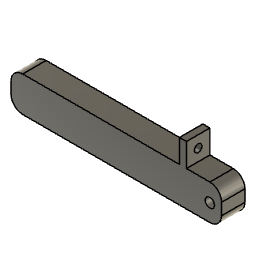
Hand_Assembly (Autodesk Fusion 360 archive; units mm, degrees)
design "Ring_Finger_Design"
Autodesk Fusion 360 part; units mm, degrees
sketch "Sketch1" plane through (0, 0, 0) normal (0, 1, 0) x (1, 0, 0)
  line L0 (0, 0) -> (90, 0)
  line L1 (90, 0) -> (90, -15)
  line L2 (90, -15) -> (0, -15)
  line L3 (0, -15) -> (0, 0)
  dimension "d1" = 90
  dimension "d2" = 15
  constraint horizontal L0
  constraint vertical L1
  constraint horizontal L2
  constraint vertical L3
  constraint coincident L0.start L3.end
  measures "d1" distance of L0.start L0.end
  measures "d2" distance of L0.start L2.end
extrude "Extrude1" add sketch "Sketch1" along normal blind 10
fillet "Fillet1" radius 5 4 edges at (0, 5, 15) (0, 5, 0) (90, 5, 15) (90, 5, 0)
sketch "Sketch2" plane through (0, 0, 0) normal (0, -1, 0) x (1, 0, 0)
  arc A0 (85, 0) -> (90, 5) centre (85, 5) ccw
  line L0 (90, 5) -> (90, 10)
  arc A1 (90, 10) -> (85, 15) centre (85, 10) ccw
  line L1 (85, 15) -> (5, 15)
  arc A2 (5, 15) -> (0, 10) centre (5, 10) ccw
  line L2 (0, 10) -> (0, 5)
  arc A3 (0, 5) -> (5, 0) centre (5, 5) ccw
  line L3 (5, 0) -> (85, 0)
  circle A4 centre (85, 7.3151) radius 2
  dimension "d7" = 4
  measures "d7" diameter of A4
extrude "Extrude2" cut sketch "Sketch2" against normal blind 28 contours A4
sketch "Sketch3" plane through (0, 0, 15) normal (0, 0, 1) x (-1, 0, 0)
  line L0 (-85, 0) -> (-85, -10)
  line L1 (-85, -10) -> (-5, -10)
  line L2 (-5, -10) -> (-5, 0)
  line L3 (-5, 0) -> (-85, 0)
  line L4 (-72, -10) -> (-75, -10)
  line L5 (-75, -10) -> (-75, 0)
  line L6 (-75, 0) -> (-72, 0)
  line L7 (-72, 0) -> (-72, -10)
  dimension "d10" = 3
  dimension "d11" = 10
  constraint horizontal L4
  constraint vertical L5
  constraint horizontal L6
  constraint vertical L7
  constraint coincident L1 L4.start
  measures "d10" distance of L4.start L4.end
  measures "d11" distance of L0 L5
extrude "Extrude3" add sketch "Sketch3" along normal blind 10 contours L1 L3 L4 L5 L6 L7
sketch "Sketch4" plane through (75, 0, 0) normal (1, 0, 0) x (0, 1, 0)
  line L0 (0, 15) -> (10, 15)
  line L1 (10, 15) -> (10, 25)
  line L2 (10, 25) -> (0, 25)
  line L3 (0, 25) -> (0, 15)
  circle A0 centre (5, 20) radius 1.625
  dimension "d14" = 3.25
  measures "d14" diameter of A0
extrude "Extrude4" cut sketch "Sketch4" against normal blind 160 contours A0

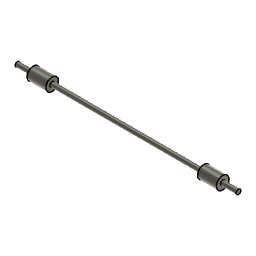
design "Connecting Rod_Hand"
Autodesk Fusion 360 part; units mm, degrees
sketch "Sketch1" plane through (0, 0, 0) normal (1, 0, 0) x (0, 1, 0)
  circle A0 centre (0, 0) radius 1.5
  dimension "d1" = 3
  constraint coincident A0.centre origin
  measures "d1" diameter of A0
extrude "Extrude1" add sketch "Sketch1" along normal blind 30
sketch "Sketch2" plane through (0, 0, 0) normal (0, 0, 1) x (1, 0, 0)
extrude "Extrude2" add 1 faces at (30, 0.567, -0.5383) along direction (1, 0, 0) blind 110
ref_plane "WorkPlane1" through (130, 0, 0) normal (1, 0, 0) x (0, 1, 0)
sketch "Sketch3" plane through (130, 0, 0) normal (1, 0, 0) x (0, 1, 0)
  circle A0 centre (0, 0) radius 4
  dimension "d7" = 8
  constraint coincident A0.centre origin
  measures "d7" diameter of A0
extrude "Extrude3" add sketch "Sketch3" against normal blind 12
ref_plane "WorkPlane2" through (10, 0, 0) normal (1, 0, 0) x (0, 1, 0)
sketch "Sketch4" plane through (10, 0, 0) normal (1, 0, 0) x (0, 1, 0)
  circle A0 centre (0, 0) radius 4
  constraint coincident A0.centre origin
extrude "Extrude4" add sketch "Sketch4" along normal blind 12

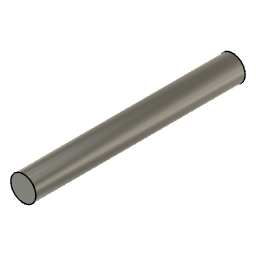
design "Connecting_Rod_Finger_Joint"
Autodesk Fusion 360 part; units mm, degrees
sketch "Sketch1" plane through (0, 0, 0) normal (0, 1, 0) x (1, 0, 0)
  circle A0 centre (0, 0) radius 1.5
  dimension "d1" = 3
  constraint coincident A0.centre origin
  measures "d1" diameter of A0
extrude "Extrude1" add sketch "Sketch1" along normal blind 25

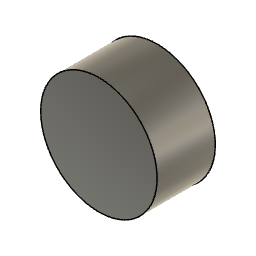
design "Rod_Caps"
Autodesk Fusion 360 part; units mm, degrees
sketch "Sketch1" plane through (0, 0, 0) normal (0, 1, 0) x (1, 0, 0)
  circle A0 centre (0, 0) radius 5
  dimension "d1" = 10
  constraint coincident A0.centre origin
  measures "d1" diameter of A0
extrude "Extrude1" add sketch "Sketch1" along normal blind 5
sketch "Sketch2" plane through (0, 5, 0) normal (0, 1, 0) x (-1, 0, 0)
  circle A0 centre (0, 0) radius 5
  circle A1 centre (0, 0) radius 1.625
  dimension "d4" = 3.25
  constraint concentric A0 A1
  measures "d4" diameter of A1
extrude "Extrude2" cut sketch "Sketch2" against normal blind 3 contours A1

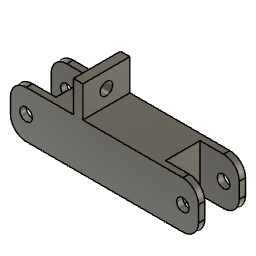
design "Main_Finger_Joint"
Autodesk Fusion 360 part; units mm, degrees
sketch "Sketch1" plane through (0, 0, 0) normal (0, 1, 0) x (1, 0, 0)
  line L0 (0, 0) -> (60, 0)
  line L1 (60, 0) -> (60, -15)
  line L2 (60, -15) -> (0, -15)
  line L3 (0, -15) -> (0, 0)
  dimension "d1" = 60
  dimension "d2" = 15
  constraint horizontal L0
  constraint vertical L1
  constraint horizontal L2
  constraint vertical L3
  constraint coincident L0.start L3.end
  measures "d1" distance of L0.start L0.end
  measures "d2" distance of L0.start L2.end
extrude "Extrude1" add sketch "Sketch1" along normal blind 15
sketch "Sketch2" plane through (0, 0, 15) normal (0, 0, 1) x (-1, 0, 0)
  line L0 (0, 0) -> (-60, 0)
  line L1 (-60, 0) -> (-60, -15)
  line L2 (-60, -15) -> (0, -15)
  line L3 (0, -15) -> (0, 0)
  line L4 (0, -13) -> (-12.5, -13)
  line L5 (-12.5, -13) -> (-12.5, -2)
  line L6 (-12.5, -2) -> (0, -2)
  line L7 (0, -2) -> (0, -13)
  line L8 (-47.5, -15) -> (-47.5, 0)
  line L9 (-47.5, -13) -> (-60, -13)
  line L10 (-47.5, -2) -> (-47.5, -13)
  line L11 (-60, -13) -> (-60, -2)
  line L12 (-60, -2) -> (-47.5, -2)
  point P0 (-47.5, 0)
  dimension "d5" = 12.5
  dimension "d6" = 11
  dimension "d7" = 2
  dimension "d8" = 12.5
  dimension "d9" = 11
  constraint horizontal L4
  constraint vertical L5
  constraint horizontal L6
  constraint vertical L7
  constraint coincident L3 L4.start
  constraint horizontal L9
  constraint vertical L11
  constraint horizontal L12
  constraint vertical L10
  constraint coincident L9.start L8
  measures "d5" distance of L4.start L4.end
  measures "d6" distance of L4.start L6.end
  measures "d7" distance of L2 L4
  measures "d8" distance of L9.start L9.end
  measures "d9" distance of L9.start L10.start
extrude "Extrude2" cut sketch "Sketch2" against normal blind 70 contours L3 L4 L5 L6 L7 | L1 L8 L9 L10 L11 L12
fillet "Fillet1" radius 5 3 edges at (0, 14, 15) (0, 1, 15) (60, 14, 15)
fillet "Fillet2" radius 5 2 edges at (0, 1, 0) (0, 14, 0)
fillet "Fillet3" radius 5 3 edges at (60, 1, 15) (60, 14, 0) (60, 1, 0)
sketch "Sketch3" plane through (0, 0, 0) normal (0, -1, 0) x (1, 0, 0)
  arc A0 (55, 0) -> (60, 5) centre (55, 5) ccw
  line L0 (60, 5) -> (60, 10)
  arc A1 (60, 10) -> (55, 15) centre (55, 10) ccw
  line L1 (55, 15) -> (5, 15)
  arc A2 (5, 15) -> (0, 10) centre (5, 10) ccw
  line L2 (0, 10) -> (0, 5)
  arc A3 (0, 5) -> (5, 0) centre (5, 5) ccw
  line L3 (5, 0) -> (55, 0)
  circle A4 centre (4.978, 7.5) radius 2
  circle A5 centre (55.0076, 7.5) radius 2
  dimension "d18" = 4
  dimension "d19" = 4
  measures "d18" diameter of A4
  measures "d19" diameter of A5
extrude "Extrude3" cut sketch "Sketch3" against normal blind 35 contours A4 | A5
sketch "Sketch4" plane through (0, 0, 15) normal (0, 0, 1) x (-1, 0, 0)
  line L0 (-55, 0) -> (-55, -2)
  line L1 (-55, -2) -> (-47.5, -2)
  line L2 (-47.5, -2) -> (-47.5, -13)
  line L3 (-47.5, -13) -> (-55, -13)
  line L4 (-55, -13) -> (-55, -15)
  line L5 (-55, -15) -> (-5, -15)
  line L6 (-5, -15) -> (-5, -13)
  line L7 (-5, -13) -> (-12.5, -13)
  line L8 (-12.5, -13) -> (-12.5, -2)
  line L9 (-12.5, -2) -> (-5, -2)
  line L10 (-5, -2) -> (-5, 0)
  line L11 (-5, 0) -> (-55, 0)
  line L12 (-20.0966, -15) -> (-23.0966, -15)
  line L13 (-23.0966, -15) -> (-23.0966, 0)
  line L14 (-23.0966, 0) -> (-20.0966, 0)
  line L15 (-20.0966, 0) -> (-20.0966, -15)
  dimension "d22" = 3
  constraint horizontal L12
  constraint vertical L13
  constraint horizontal L14
  constraint vertical L15
  constraint coincident L5 L12.start
  measures "d22" distance of L12.start L12.end
extrude "Extrude4" add sketch "Sketch4" along normal blind 10 contours L5 L11 L12 L13 L14 L15
sketch "Sketch5" plane through (23.0966, 0, 0) normal (1, 0, 0) x (0, 1, 0)
  line L0 (0, 15) -> (15, 15)
  line L1 (15, 15) -> (15, 25)
  line L2 (15, 25) -> (0, 25)
  line L3 (0, 25) -> (0, 15)
  circle A0 centre (7.5, 19.9253) radius 2
  dimension "d25" = 4
  measures "d25" diameter of A0
extrude "Extrude5" cut sketch "Sketch5" against normal blind 28 contours A0

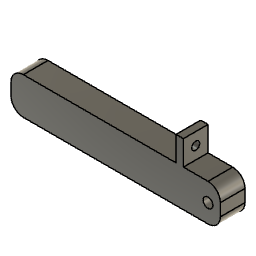
design "Index_Finger_Design"
Autodesk Fusion 360 part; units mm, degrees
sketch "Sketch1" plane through (0, 0, 0) normal (0, 1, 0) x (1, 0, 0)
  line L0 (0, 0) -> (85, 0)
  line L1 (85, 0) -> (85, -15)
  line L2 (85, -15) -> (0, -15)
  line L3 (0, -15) -> (0, 0)
  dimension "d1" = 85
  dimension "d2" = 15
  constraint horizontal L0
  constraint vertical L1
  constraint horizontal L2
  constraint vertical L3
  constraint coincident L0.start L3.end
  measures "d1" distance of L0.start L0.end
  measures "d2" distance of L0.start L2.end
extrude "Extrude1" add sketch "Sketch1" along normal blind 10
fillet "Fillet1" radius 5 4 edges at (0, 5, 15) (0, 5, 0) (85, 5, 15) (85, 5, 0)
sketch "Sketch2" plane through (0, 0, 15) normal (0, 0, 1) x (-1, 0, 0)
  line L0 (-80, 0) -> (-80, -10)
  line L1 (-80, -10) -> (-5, -10)
  line L2 (-5, -10) -> (-5, 0)
  line L3 (-5, 0) -> (-80, 0)
  line L4 (-67, -10) -> (-70, -10)
  line L5 (-70, -10) -> (-70, 0)
  line L6 (-70, 0) -> (-67, 0)
  line L7 (-67, 0) -> (-67, -10)
  dimension "d7" = 3
  dimension "d8" = 10
  constraint horizontal L4
  constraint vertical L5
  constraint horizontal L6
  constraint vertical L7
  constraint coincident L1 L4.start
  measures "d7" distance of L4.start L4.end
  measures "d8" distance of L0 L5
extrude "Extrude2" add sketch "Sketch2" along normal blind 10 contours L1 L3 L4 L5 L6 L7
sketch "Sketch3" plane through (0, 0, 0) normal (0, -1, 0) x (1, 0, 0)
  arc A0 (80, 0) -> (85, 5) centre (80, 5) ccw
  line L0 (85, 5) -> (85, 10)
  arc A1 (85, 10) -> (80, 15) centre (80, 10) ccw
  line L1 (80, 15) -> (70, 15)
  line L2 (70, 15) -> (70, 25)
  line L3 (70, 25) -> (67, 25)
  line L4 (67, 25) -> (67, 15)
  line L5 (67, 15) -> (5, 15)
  arc A2 (5, 15) -> (0, 10) centre (5, 10) ccw
  line L6 (0, 10) -> (0, 5)
  arc A3 (0, 5) -> (5, 0) centre (5, 5) ccw
  line L7 (5, 0) -> (80, 0)
  circle A4 centre (80, 7.4726) radius 2
  dimension "d11" = 4
  measures "d11" diameter of A4
extrude "Extrude3" cut sketch "Sketch3" against normal blind 13 contours A4
sketch "Sketch4" plane through (70, 0, 0) normal (1, 0, 0) x (0, 1, 0)
  line L0 (0, 15) -> (10, 15)
  line L1 (10, 15) -> (10, 25)
  line L2 (10, 25) -> (0, 25)
  line L3 (0, 25) -> (0, 15)
  circle A0 centre (5, 20.0248) radius 1.625
  dimension "d14" = 3.25
  measures "d14" diameter of A0
extrude "Extrude4" cut sketch "Sketch4" against normal blind 56 contours A0

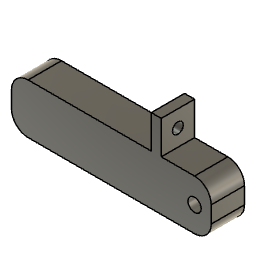
design "Pinky_Finger_Design"
Autodesk Fusion 360 part; units mm, degrees
sketch "Sketch1" plane through (0, 0, 0) normal (0, 1, 0) x (1, 0, 0)
  line L0 (0, 0) -> (60, 0)
  line L1 (60, 0) -> (60, -15)
  line L2 (60, -15) -> (0, -15)
  line L3 (0, -15) -> (0, 0)
  dimension "d1" = 60
  dimension "d2" = 15
  constraint horizontal L0
  constraint vertical L1
  constraint horizontal L2
  constraint vertical L3
  constraint coincident L0.start L3.end
  measures "d1" distance of L0.start L0.end
  measures "d2" distance of L0.start L2.end
extrude "Extrude1" add sketch "Sketch1" along normal blind 10
fillet "Fillet1" radius 5 4 edges at (0, 5, 15) (0, 5, 0) (60, 5, 15) (60, 5, 0)
sketch "Sketch2" plane through (0, 0, 0) normal (0, -1, 0) x (1, 0, 0)
  arc A0 (55, 0) -> (60, 5) centre (55, 5) ccw
  line L0 (60, 5) -> (60, 10)
  arc A1 (60, 10) -> (55, 15) centre (55, 10) ccw
  line L1 (55, 15) -> (5, 15)
  arc A2 (5, 15) -> (0, 10) centre (5, 10) ccw
  line L2 (0, 10) -> (0, 5)
  arc A3 (0, 5) -> (5, 0) centre (5, 5) ccw
  line L3 (5, 0) -> (55, 0)
  circle A4 centre (54.9991, 7.5) radius 2
  dimension "d7" = 4
  measures "d7" diameter of A4
extrude "Extrude2" cut sketch "Sketch2" against normal blind 150 contours A4
sketch "Sketch3" plane through (0, 0, 15) normal (0, 0, 1) x (-1, 0, 0)
  line L0 (-55, 0) -> (-55, -10)
  line L1 (-55, -10) -> (-5, -10)
  line L2 (-5, -10) -> (-5, 0)
  line L3 (-5, 0) -> (-55, 0)
  line L4 (-42, -10) -> (-45, -10)
  line L5 (-45, -10) -> (-45, 0)
  line L6 (-45, 0) -> (-42, 0)
  line L7 (-42, 0) -> (-42, -10)
  dimension "d10" = 3
  dimension "d11" = 10
  dimension "d12" = 10
  constraint horizontal L4
  constraint vertical L5
  constraint horizontal L6
  constraint vertical L7
  constraint coincident L1 L4.start
  measures "d10" distance of L4.start L4.end
  measures "d11" distance of L4.start L6.end
  measures "d12" distance of L0 L5
extrude "Extrude3" add sketch "Sketch3" along normal blind 10 contours L1 L3 L4 L5 L6 L7
sketch "Sketch4" plane through (45, 0, 0) normal (1, 0, 0) x (0, 1, 0)
  line L0 (0, 15) -> (10, 15)
  line L1 (10, 15) -> (10, 25)
  line L2 (10, 25) -> (0, 25)
  line L3 (0, 25) -> (0, 15)
  circle A0 centre (5, 20) radius 1.625
  dimension "d15" = 3.25
  measures "d15" diameter of A0
extrude "Extrude4" cut sketch "Sketch4" against normal blind 52 contours A0

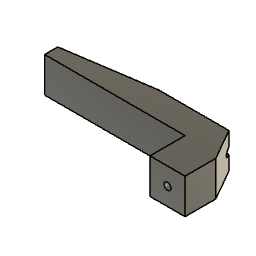
design "Thumb_Initial_Design"
Autodesk Fusion 360 part; units mm, degrees
sketch "Sketch1" plane through (0, 0, 0) normal (0, 1, 0) x (1, 0, 0)
  line L0 (0, 0) -> (20, 0)
  line L1 (20, 0) -> (20, -20)
  line L2 (20, -20) -> (0, -20)
  line L3 (0, -20) -> (0, 0)
  dimension "d1" = 20
  dimension "d2" = 20
  constraint horizontal L0
  constraint vertical L1
  constraint horizontal L2
  constraint vertical L3
  constraint coincident L0.start L3.end
  measures "d1" distance of L0.start L0.end
  measures "d2" distance of L0.start L2.end
extrude "Extrude1" add sketch "Sketch1" along normal blind 20
sketch "Sketch2" plane through (0, 20, 0) normal (0, 1, 0) x (-1, 0, 0)
  line L0 (0, 20) -> (-20, 20)
  line L1 (-20, 20) -> (-20, 0)
  line L2 (-20, 0) -> (0, 0)
  line L3 (0, 0) -> (0, 20)
  line L4 (-20, 0) -> (80, 0)
  line L5 (80, 0) -> (80, 20)
  line L6 (80, 20) -> (-20, 20)
  line L7 (-20, 20) -> (-20, 0)
  dimension "d5" = 100
  constraint horizontal L4
  constraint vertical L5
  constraint horizontal L6
  constraint vertical L7
  constraint coincident L1.end L2.start
  measures "d5" distance of L1.end L4.end
extrude "Extrude2" add sketch "Sketch2" along normal blind 15
sketch "Sketch3" plane through (0, 0, 20) normal (0, 0, 1) x (-1, 0, 0)
  line L0 (0, 0) -> (-20, 0)
  line L1 (-20, 0) -> (-20, -35)
  line L2 (-20, -35) -> (80, -35)
  line L3 (80, -35) -> (80, -20)
  line L4 (80, -20) -> (0, -20)
  line L5 (0, -20) -> (0, 0)
  line L6 (80, -27.5) -> (30, -35)
  line L7 (80, -27.5) -> (80, -35)
  line L8 (-10, -35) -> (-20, -17.5)
  line L9 (-20, -17.5) -> (-20, -35)
  line L10 (-10, -35) -> (-20, -35)
  line L11 (80, -35) -> (30, -35)
  constraint midpoint L3 L6.start
  constraint midpoint L2 L6.end
  constraint coincident L2.end L3.start
  constraint coincident L2 L8.start
  constraint midpoint L1 L8.end
  constraint coincident L1.end L2.start
  constraint perpendicular L1 L10
extrude "Extrude3" cut sketch "Sketch3" against normal blind 50 contours L1 L2 L8 L9 L10 | L2 L3 L6 L7 L11
sketch "Sketch4" plane through (0, 0, 0) normal (0, -1, 0) x (1, 0, 0)
  line L0 (20, 20) -> (0, 20)
  line L1 (0, 20) -> (0, 0)
  line L2 (0, 0) -> (20, 0)
  line L3 (20, 0) -> (20, 20)
  circle A0 centre (10, 10) radius 2
  dimension "d10" = 4
  measures "d10" diameter of A0
extrude "Extrude4" cut sketch "Sketch4" against normal blind 40 contours A0
